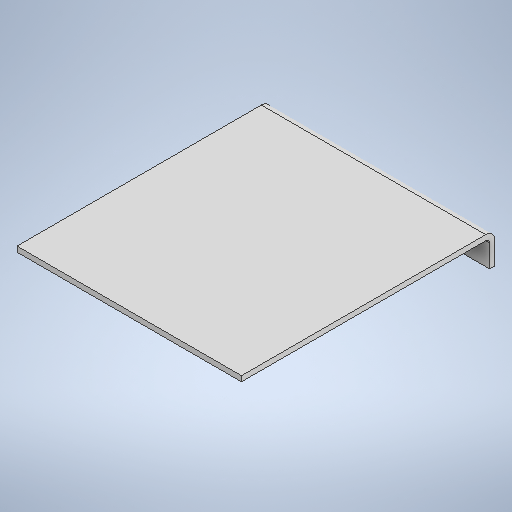
# Autodesk Inventor part: TS_V1_Fallmagazin_Blech_int
Saved by Autodesk Inventor 2025.2 (Build 292293000, 293)
## iProperties
Created: 2025-06-13
Part Number: TS_V1_Fallmagazin_Blech_int
Material: Generisch
Document SubType Name: Modeling
Designer: tino
Density: 1 g/cm^3
Appearance: Vorgabe
Author: tino
Autodesk Inventor part; units mm, degrees
ref_plane "YZ Plane" through (0, 0, 0) normal (1, 0, 0) x (0, 1, 0)
ref_plane "XZ Plane" through (0, 0, 0) normal (0, 1, 0) x (-1, 0, 0)
ref_plane "XY Plane" through (0, 0, 0) normal (0, 0, 1) x (1, 0, 0)
sketch "Skizze2" plane through (0, 0, 0) normal (1, 0, 0) x (0, 1, 0)
  line L0 (-189.6555, 61.2009) -> (-93.6555, 61.2009)
  line L1 (-93.6555, 61.2009) -> (-93.6555, 59.2009)
  line L2 (-93.6555, 59.2009) -> (-189.6555, 59.2009)
  line L3 (-189.6555, 59.2009) -> (-189.6555, 61.2009)
  line L4 (-93.6555, 61.2009) -> (-95.6555, 61.2009)
  line L5 (-95.6555, 61.2009) -> (-95.6555, 49.2009)
  line L6 (-95.6555, 49.2009) -> (-93.6555, 49.2009)
  line L7 (-93.6555, 49.2009) -> (-93.6555, 61.2009)
  point P0 (0, 0)
  point P1 (-95.6555, 59.2009)
  dimension "d0" = 96
  dimension "d1" = 2
  dimension "d2" = 2
  dimension "d3" = 12
  constraints: 16 end point, 4 parallel, 2 horizontal, 2 perpendicular
  measures "d0" distance of L1.end L2.end
  measures "d1" distance of L0.end L1.end
  measures "d2" distance of L6.end L5.end
  measures "d3" distance of L5.end L4.end
extrude "Extrusion1" add sketch "Skizze2" along normal blind 85
sketch "Skizze3" plane through (0, -93.6555, 61.2009) normal (0, 1, 0) x (1, 0, 0)
  line L0 (0, 12) -> (85, 12) projected
  line L1 (0, 0) -> (85, 0) projected
  line L2 (85, 12) -> (85, 0) projected
  line L3 (0, 12) -> (0, 0) projected
  point P0 (0, 61.2009)
  point P1 (75, 7.75)
  point P2 (10, 7.75)
  dimension "d6" = 12
  dimension "d8" = 10
  dimension "d9" = 10
  dimension "d20" = 4.25
  constraints: 1 horizontal alignment
  measures "d6" distance between parallel lines of L0 L1
  measures "d8" distance from line of point (75, 7.75) L2
  measures "d9" distance from line of L3 point (10, 7.75)
  measures "d20" distance from line of L0 point (75, 7.75)
hole "Bohrung1" at (75, -93.6555, 53.4509) at (10, -93.6555, 53.4509) direction (0, -1, 0) diameter 4.2 end through all
fillet "Rundung2" radius 3.5 1 edges at (42.5, -93.6555, 61.2009)
fillet "Rundung3" radius 1.5 1 edges at (42.5, -95.6555, 59.2009)
